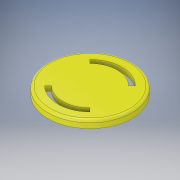
# Autodesk Inventor part: circularholder
Saved by Autodesk Inventor 2019 (Build 230136000, 136)
## iProperties
Created: 2019-02-20
Part Number: circularholder
Material: PET Plastic
Document SubType Name: Modeling
Designer: jmc
Density: 1.541 g/cm^3
Appearance: Yellow
Author: jmc
Autodesk Inventor part; units mm, degrees
ref_plane "YZ Plane" through (0, 0, 0) normal (1, 0, 0) x (0, 1, 0)
ref_plane "XZ Plane" through (0, 0, 0) normal (0, 1, 0) x (-1, 0, 0)
ref_plane "XY Plane" through (0, 0, 0) normal (0, 0, 1) x (1, 0, 0)
sketch "Sketch1" plane through (0, 0, 0) normal (0, 1, 0) x (-1, 0, 0)
  circle A0 centre (0, 0) radius 17
  dimension "d0" = 34
  constraints: 1 centre point, 1 coincident
  measures "d0" diameter of A0
extrude "Extrusion1" add sketch "Sketch1" along normal blind 2
sketch "Sketch2" plane through (0, 0, 0) normal (0, -1, 0) x (1, 0, 0)
  circle A0 centre (0, 0) radius 17 projected
  circle A1 centre (0, 0) radius 15
  dimension "d3" = 2
  constraints: 1 centre point
  measures "d3" radial gap between concentric circles of A0 A1
extrude "Extrusion2" add sketch "Sketch2" along normal blind 1
sketch "Sketch3" plane through (0, 2, 0) normal (0, 1, 0) x (1, 0, 0)
  circle A0 centre (0, 0) radius 17 projected
  arc A1 (-9.1924, -9.1924) -> (9.1924, -9.1924) centre (0, 0) ccw
  arc A2 (-7.7782, -7.7782) -> (7.7782, -7.7782) centre (0, 0) ccw
  line L0 (0, 0) -> (-9.1924, -9.1924) construction
  line L1 (0, 0) -> (9.1924, -9.1924) construction
  line L2 (-9.1924, -9.1924) -> (-7.7782, -7.7782)
  line L3 (7.7782, -7.7782) -> (9.1924, -9.1924)
  dimension "d6" = 4
  dimension "d7" = 2
  constraints: 8 end point, 4 point on circle, 2 centre point, 2 point on line, 1 collinear
  measures "d6" radial gap between concentric circles of A0 A1
  measures "d7" radial gap between concentric circles of A1 A2
extrude "Extrusion3" cut sketch "Sketch3" against normal through all contours L2 A2 L3 A1
mirror "Mirror1" about plane through (0, 0, 0) normal (0, 0, 1) of "Extrusion3"
fillet "Fillet1" radius 1 1 edges at (17, 2, 0)
body "Solid1"
